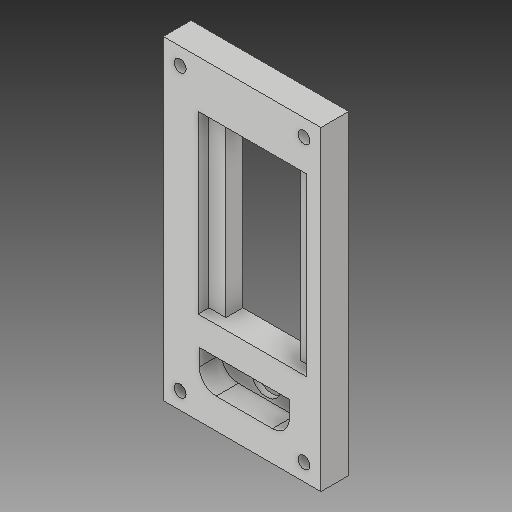
# Autodesk Inventor part: FrontPanel
Saved by Autodesk Inventor 2018 (Build 220112000, 112)
## iProperties
Created: 2020-03-31
Part Number: FrontPanel
Material: Generic
Document SubType Name: Modeling
Designer: emile
Density: 1 g/cm^3
Appearance: Default
Mass: 156.797 g
Surface Area: 387.8 cm^2
Volume: 156.797 cm^3
Author: emile
Autodesk Inventor part; units mm, degrees
ref_plane "YZ Plane" through (0, 0, 0) normal (1, 0, 0) x (0, 1, 0)
ref_plane "XZ Plane" through (0, 0, 0) normal (0, 1, 0) x (-1, 0, 0)
ref_plane "XY Plane" through (0, 0, 0) normal (0, 0, 1) x (1, 0, 0)
sketch "Sketch1" plane through (0, 0, 0) normal (0, 0, 1) x (1, 0, 0)
  line L0 (44.45, -88.9) -> (-44.45, -88.9)
  line L1 (-44.45, -88.9) -> (-44.45, 88.9)
  line L2 (-44.45, 88.9) -> (44.45, 88.9)
  line L3 (44.45, 88.9) -> (44.45, -88.9)
  line L4 (44.45, -88.9) -> (-44.45, 88.9) construction
  line L5 (-44.45, -88.9) -> (44.45, 88.9) construction
  line L6 (26.659, 62.23) -> (-15.251, 62.23)
  line L7 (-15.251, 62.23) -> (-15.251, -36.83)
  line L8 (-15.251, -36.83) -> (26.659, -36.83)
  line L9 (26.659, -36.83) -> (26.659, 62.23)
  line L10 (5.704, 62.23) -> (5.704, -36.83) construction
  line L11 (36.184, -36.83) -> (-24.776, -36.83)
  line L12 (-24.776, -36.83) -> (-24.776, 62.23)
  line L13 (-24.776, 62.23) -> (36.184, 62.23)
  line L14 (36.184, 62.23) -> (36.184, -36.83)
  line L15 (36.184, -36.83) -> (-24.776, 62.23) construction
  line L16 (-24.776, -36.83) -> (36.184, 62.23) construction
  point P0 (0, 0)
  point P1 (5.704, 12.7)
  dimension "d0" = 88.9
  dimension "d1" = 177.8
  dimension "d2" = 62.23
  dimension "d3" = 99.06
  dimension "d4" = 41.91
  dimension "d6" = 26.659
  dimension "d16" = 99.06
  dimension "d17" = 60.96
  constraints: 34 end point, 7 midpoint, 6 parallel, 3 horizontal, 3 perpendicular
  measures "d0" distance of L1.end L2.end
  measures "d1" distance of L2.end L0.start
  measures "d2" distance from line of point (0, 0) L6
  measures "d3" distance of L8.end L6.start
  measures "d4" distance of L6.start L6.end
  measures "d6" distance from line of point (0, 0) L9
  measures "d16" distance of L13.end L11.start
  measures "d17" distance between parallel lines of L14 L12
extrude "Extrusion1" add sketch "Sketch1" against normal blind 3.175 contours L0 L1 L2 L3 | L13 L14 L11 L9 | L7 L11 L12 L13
ref_plane "Work Plane1" through (-44.45, 0, 0) normal (0, 1, 0) x (1, 0, 0)
ref_plane "Work Plane2" through (0, -88.9, 0) normal (1, 0, 0) x (0, 0, -1)
ref_plane "Work Plane3" through (-15.251, 12.7, 0) normal (0, 1, 0) x (1, 0, 0)
ref_plane "Work Plane4" through (5.704, -36.83, 0) normal (1, 0, 0) x (0, 0, -1)
sketch "Sketch2" plane through (0, 0, -3.175) normal (0, 0, -1) x (-1, 0, 0)
  point P0 (-1.25, -62.3)
hole "Hole1" at (1.25, -62.3, -3.175) direction (0, 0, 1) diameter 16.6675 depth 3.175
extrude "Extrusion2" add sketch "Sketch1" along normal blind 6.4008 contours L13 L14 L11 L9 | L7 L11 L12 L13
sketch "Sketch3" plane through (0, 0, 0) normal (0, 0, 1) x (1, 0, 0)
  line L0 (44.45, -88.9) -> (-44.45, -88.9) projected
  line L1 (44.45, 88.9) -> (44.45, -88.9) projected
  line L2 (-44.45, 88.9) -> (44.45, 88.9) projected
  line L3 (-44.45, -88.9) -> (-44.45, 88.9) projected
  circle A0 centre (1.25, -62.3) radius 8.3337 projected
  line L4 (26.659, 62.23) -> (36.184, 62.23) projected
  line L5 (36.184, 62.23) -> (36.184, -36.83) projected
  line L6 (36.184, -36.83) -> (26.659, -36.83) projected
  line L7 (26.659, -36.83) -> (-15.251, -36.83) projected
  line L8 (-15.251, -36.83) -> (-24.776, -36.83) projected
  line L9 (-24.776, -36.83) -> (-24.776, 62.23) projected
  line L10 (-24.776, 62.23) -> (-15.251, 62.23) projected
  line L11 (-15.251, 62.23) -> (26.659, 62.23) projected
  line L12 (26.65, -52.775) -> (-24.15, -52.775)
  line L13 (-24.15, -52.775) -> (-24.15, -71.825)
  line L14 (-24.15, -71.825) -> (26.65, -71.825)
  line L15 (26.65, -71.825) -> (26.65, -52.775)
  circle A1 centre (19.35, -61.6904) radius 1.5875
  point P0 (0, 0)
  point P1 (26.65, -62.3)
  dimension "d20" = 25.4
  dimension "d21" = 25.4
  dimension "d22" = 19.05
  dimension "d26" = 3.175
  dimension "d29" = 0.6096
  dimension "d30" = 18.1
  constraints: 8 end point, 2 parallel, 1 centre point, 1 horizontal, 1 horizontal alignment, 1 midpoint, 1 perpendicular
  measures "d20" distance from line of A0.centre L15
  measures "d21" distance from line of L13 A0.centre
  measures "d22" distance of L14.end L12.start
  measures "d26" diameter of A1
  measures "d29" vertical distance of A0.centre A1.centre
  measures "d30" horizontal distance of A0.centre A1.centre
extrude "Extrusion3" add sketch "Sketch3" along normal blind 12.5222 contours L0 L3 L2 L1
extrude "Extrusion4" cut sketch "Sketch3" against normal through all contours A1
fillet "Fillet1" radius 9.525 2 edges at (26.65, -71.825, 6.2611) (-24.15, -71.825, 6.2611)
sketch "Sketch4" plane through (0, 0, -3.175) normal (0, 0, -1) x (-1, 0, 0)
  point P0 (-34.925, -79.375)
  point P1 (-34.925, 79.375)
  point P2 (34.925, 79.375)
  point P3 (34.925, -79.375)
hole "Hole3" at (34.925, -79.375, -3.175) at (34.925, 79.375, -3.175) at (-34.925, 79.375, -3.175) at (-34.925, -79.375, -3.175) direction (0, 0, 1) diameter 6.7564 depth 15.6972
body "Solid1"
